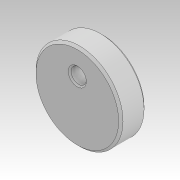
# Autodesk Inventor part: TestCam
Saved by Autodesk Inventor 2020 (Build 240168000, 168)
## iProperties
Created: 2021-05-17
Part Number: TestCam
Material: Generic
Document SubType Name: Modeling
Designer: DDeGo
Density: 1 g/cm^3
Appearance: Default
Author: DDeGo
Autodesk Inventor part; units mm, degrees
ref_plane "YZ Plane" through (0, 0, 0) normal (1, 0, 0) x (0, 1, 0)
ref_plane "XZ Plane" through (0, 0, 0) normal (0, 1, 0) x (-1, 0, 0)
ref_plane "XY Plane" through (0, 0, 0) normal (0, 0, 1) x (1, 0, 0)
sketch "Sketch1" plane through (0, 0, 0) normal (0, 0, 1) x (1, 0, 0)
  circle A0 centre (0, 0) radius 6
  dimension "d0" = 12
  constraints: 1 centre point, 1 coincident
  measures "d0" diameter of A0
extrude "Extrusion1" add sketch "Sketch1" along normal mid plane 3.5
sketch "Sketch2" plane through (0, 0, 1.75) normal (0, 0, 1) x (1, 0, 0)
  circle A0 centre (0, 2.5) radius 1.05
  line L0 (0, 2.5) -> (0, 0) construction
  dimension "d3" = 2.1
  dimension "d4" = 2.5
  constraints: 2 end point, 1 centre point, 1 vertical
  measures "d3" diameter of A0
  measures "d4" distance of L0.start L0.end
extrude "Extrusion2" add sketch "Sketch2" along normal blind 15 and the other way blind 8.25
chamfer "Chamfer1" distance 0.3 angle 45 2 edges at (-6, 0, 1.75) (-6, 0, -1.75)
sketch "Sketch4" plane through (0, 2.5, -6.5) normal (0, 0, -1) x (-1, 0, 0)
  circle A0 centre (0, 0) radius 1.05 projected
  point P0 (0, -2.5)
extrude "Extrusion4" cut sketch "Sketch4" against normal through all
sketch "Sketch5" plane through (0, 0, 0) normal (1, 0, 0) x (0, 1, 0)
  line L0 (3.55, -1.75) -> (1.45, -1.75) construction
  line L1 (2.5, -1.75) -> (2.5, -5.85) construction
  line L2 (2.5, -6.85) -> (4.8, -6.85)
  line L3 (4.8, -6.85) -> (5, -6.65)
  line L4 (5, -6.65) -> (5, -4.55)
  line L5 (5, -4.55) -> (5.15, -4.55)
  line L6 (5.15, -4.55) -> (5.15, -4.4)
  line L7 (5.15, -4.4) -> (4.2, -4.05)
  line L8 (4.2, -4.05) -> (4.2, -1.75)
  line L9 (4.2, -1.75) -> (3.55, -1.75)
  line L10 (3.55, -1.75) -> (3.55, -5.85)
  line L11 (3.55, -5.85) -> (2.5, -5.85)
  line L12 (2.5, -5.85) -> (2.5, -6.85)
  line L13 (3.55, -1.75) -> (2.5, -1.75) construction
  point P0 (0, 0)
  dimension "d17" = 2.3
  dimension "d18" = 135
  dimension "d19" = 0.2
  dimension "d20" = 2.5
  dimension "d21" = 0.15
  dimension "d22" = 0.15
  dimension "d23" = 2.3
  dimension "d24" = 1.7
  dimension "d25" = 2.8
  dimension "d26" = 1
  constraints: 26 end point, 6 perpendicular, 4 parallel, 3 vertical, 2 collinear, 1 midpoint
  measures "d17" distance between parallel lines of L2 L5
  measures "d18" angle of L4 L3
  measures "d19" distance from line of L2.end L4
  measures "d20" distance between parallel lines of L1 L4
  measures "d21" distance of L4.end L5.end
  measures "d22" distance of L5.end L6.end
  measures "d23" distance of L7.end L8.end
  measures "d24" distance between parallel lines of L1 L8
  measures "d25" distance between parallel lines of L9 L5
  measures "d26" distance between parallel lines of L2 L11
revolve "Revolution1" [suppressed]
fillet "Fillet1" [suppressed]
chamfer "Chamfer2" distance 0.2 angle 45 2 edges at (1.05, 2.5, 1.75) (1.05, 2.5, -1.75)
sketch "Sketch6" plane through (0, 2.5, -2.8) normal (0, 0, -1) x (-1, 0, 0)
  circle A0 centre (0, -1) radius 3.5
  circle A1 centre (0, 0) radius 2.5 projected
  circle A2 centre (0, 0) radius 2.65 projected
  line L0 (0, 0) -> (0, -1) construction
  point P0 (0, -2.5)
  point P1 (1.5983, 2.1137)
  point P2 (-1.5983, 2.1137)
  dimension "d32" = 1
  constraints: 2 end point, 1 centre point, 1 vertical, 1 vertical alignment, 1 other
  measures "d32" distance of L0.start L0.end
extrude "Extrusion5" [suppressed]
sketch "Sketch7" plane through (0, 0, 0) normal (0, 0, 1) x (1, 0, 0)
  circle A0 centre (0, 2.5) radius 1.05 projected
  circle A1 centre (-1.05, 2.5) radius 0.1
  line L0 (-1.05, 2.5) -> (0, 2.5) construction
  circle A2 centre (0.525, 1.5907) radius 0.1
  circle A3 centre (0.525, 3.4093) radius 0.1
  point P0 (0, 0)
  dimension "d35" = 0.2
  dimension "d38" = 360
  constraints: 3 centre point, 2 end point, 1 horizontal, 1 horizontal alignment, 8 other
  measures "d35" diameter of A1
extrude "Extrusion6" add sketch "Sketch7" along normal mid plane 1 contours A3 A0 | A0 A3 | A2 A0 | A0 A2 | A1 A0 | A0 A1
chamfer "Chamfer3" distance 0.1 angle 45 8 edges at (-0.9776, 2.431, 0.5) (-0.9776, 2.569, 0.5) (-0.9776, 2.431, -0.5) (-0.9776, 2.569, -0.5) (0.475, 3.3227, 0.5) (0.475, 3.3227, -0.5) (0.475, 1.6773, 0.5) (0.475, 1.6773, -0.5)
fillet "Fillet2" radius 0.3 8 edges at (-0.9776, 2.431, 0.4001) (-0.9776, 2.569, 0.4001) (-0.9776, 2.431, -0.4001) (-0.9776, 2.569, -0.4001) (0.475, 1.6773, 0.4001) (0.475, 1.6773, -0.4001) (0.475, 3.3227, 0.4001) (0.475, 3.3227, -0.4001)
body "Solid1"
